Fenstergitter_v3 (Autodesk Fusion 360 design; units mm, degrees)
Autodesk Fusion 360 part; units mm, degrees
sketch "Skizze1" plane through (0, 0, 0) normal (0, 1, 0) x (1, 0, 0)
  line L0 (0, 0) -> (10, 0)
  line L1 (10, 0) -> (10, 28.5)
  line L2 (10, 28.5) -> (0, 28.5)
  line L3 (0, 28.5) -> (0, 0)
  line L4 (3.5, 9.5) -> (3.5, 3.5)
  arc A0 (3.5, 3.5) -> (6.5, 3.5) centre (5, 3.5) ccw
  line L5 (6.5, 3.5) -> (6.5, 9.5)
  arc A1 (6.5, 9.5) -> (3.5, 9.5) centre (5, 9.5) ccw
  line L6 (3.5, 21.5) -> (3.5, 15.5)
  line L7 (6.5, 15.5) -> (6.5, 21.5)
  arc A2 (6.5, 21.5) -> (3.5, 21.5) centre (5, 21.5) ccw
  arc A3 (3.5, 15.5) -> (6.5, 15.5) centre (5, 15.5) ccw
  dimension "d1" = 10
  dimension "d2" = 28.5
  dimension "d3" = 3
  dimension "d4" = 6
  dimension "d5" = 5
  dimension "d6" = 3.5
  dimension "d7" = 3
  dimension "d8" = 6
  dimension "d9" = 12
  constraint horizontal L0
  constraint vertical L1
  constraint horizontal L2
  constraint vertical L3
  constraint coincident L0.start L3.end
  constraint vertical L4
  constraint tangent L4 A0
  constraint tangent A0 L5
  constraint parallel L4 L5
  constraint tangent L5 A1
  constraint tangent L4 A1
  constraint vertical L6
  constraint tangent L6 A3
  constraint tangent L7 A3
  constraint parallel L6 L7
  constraint tangent L7 A2
  constraint tangent L6 A2
  measures "d1" distance of L0.start L0.end
  measures "d2" distance of L0.start L2.end
  measures "d3" distance of L4 L5
  measures "d4" distance of A0.centre A1.centre
  measures "d5" horizontal distance of L0.start A0.centre
  measures "d6" distance of L0 A0.centre
  measures "d7" distance of L6 L7
  measures "d8" distance of A3.centre A2.centre
  measures "d9" distance of A0.centre A3.centre
extrude "Extrusion1" add sketch "Skizze1" along normal blind 2
sketch "Skizze2" plane through (0, 2, 0) normal (0, 1, 0) x (-1, 0, 0)
  arc A0 (-6.5, -9.5) -> (-3.5, -9.5) centre (-5, -9.5) ccw
  line L0 (-6.5, -9.5) -> (-6.5, -3.5)
  arc A1 (-3.5, -3.5) -> (-6.5, -3.5) centre (-5, -3.5) ccw
  line L1 (-3.5, -3.5) -> (-3.5, -9.5)
  arc A2 (-3.5, -15.5) -> (-6.5, -15.5) centre (-5, -15.5) ccw
  line L2 (-3.5, -15.5) -> (-3.5, -21.5)
  arc A3 (-6.5, -21.5) -> (-3.5, -21.5) centre (-5, -21.5) ccw
  line L3 (-6.5, -21.5) -> (-6.5, -15.5)
  line L4 (0, -28.5) -> (0, 0)
  line L5 (0, 0) -> (-10, 0)
  line L6 (-10, 0) -> (-10, -28.5)
  line L7 (-10, -28.5) -> (0, -28.5)
  line L8 (-10, -28.5) -> (0, -28.5)
  line L9 (0, -28.5) -> (0, -25)
  line L10 (0, -25) -> (-10, -25)
  line L11 (-10, -25) -> (-10, -28.5)
  constraint horizontal L8
  constraint vertical L9
  constraint horizontal L10
  constraint vertical L11
  constraint coincident L4 L9.end
  constraint coincident L6.end L7.start
ref_plane "Arbeitsebene1" through (5, 18, -26.75) normal (0, 1, 0) x (-1, 0, 0)
sketch "Skizze3" plane through (5, 18, -26.75) normal (0, 1, 0) x (1, 0, 0)
ref_plane "Arbeitsebene2" through (5, 16, -6.5) normal (0, 1, 0) x (-1, 0, 0)
sketch "Skizze4" plane through (5, 16, -26.75) normal (0, 1, 0) x (1, 0, 0)
  arc A0 (1.5, -17.25) -> (-1.5, -17.25) centre (0, -17.25) ccw
  line L0 (1.5, -17.25) -> (1.5, -23.25)
  arc A1 (-1.5, -23.25) -> (1.5, -23.25) centre (0, -23.25) ccw
  line L1 (-1.5, -23.25) -> (-1.5, -17.25)
  arc A2 (-1.5, -11.25) -> (1.5, -11.25) centre (0, -11.25) ccw
  line L2 (-1.5, -11.25) -> (-1.5, -5.25)
  arc A3 (1.5, -5.25) -> (-1.5, -5.25) centre (0, -5.25) ccw
  line L3 (1.5, -5.25) -> (1.5, -11.25)
  line L4 (-5, 1.75) -> (-5, -26.75)
  line L5 (-5, -26.75) -> (5, -26.75)
  line L6 (5, -26.75) -> (5, 1.75)
  line L7 (5, 1.75) -> (-5, 1.75)
  line L8 (5, 1.75) -> (-5, 1.75)
  line L9 (-5, 1.75) -> (-5, -0.75)
  line L10 (-5, -0.75) -> (5, -0.75)
  line L11 (5, -0.75) -> (5, 1.75)
  dimension "d14" = 2.5
  constraint horizontal L8
  constraint vertical L9
  constraint horizontal L10
  constraint vertical L11
  constraint coincident L6.end L7.start
  measures "d14" distance of L6.end L10.end
loft "Erhebung1" add profiles "Skizze2", "Skizze4" section 1 contours L4 L6 L7 L8 L9 L10 L11 section 2 contours L4 L6 L7 L8 L9 L10 L11
sketch "Skizze5" plane through (0, 16, 0) normal (0, 1, 0) x (-1, 0, 0)
  line L0 (-10, -26) -> (-10, -28.5)
  line L1 (-10, -28.5) -> (0, -28.5)
  line L2 (0, -28.5) -> (0, -26)
  line L3 (0, -26) -> (-10, -26)
  line L4 (-10, -26) -> (0, -26)
  line L5 (0, -26) -> (0, -46)
  line L6 (0, -46) -> (-10, -46)
  line L7 (-10, -46) -> (-10, -26)
  dimension "d15" = 20
  constraint horizontal L4
  constraint vertical L5
  constraint horizontal L6
  constraint vertical L7
  constraint coincident L0.start L3.end
  measures "d15" distance of L0.start L6.end
extrude "Extrusion2" add sketch "Skizze5" along normal blind 1.2
fillet "Abrundung1" radius 0.3 19 faces at (4.9626, 0, -26.6653) (10, 6, -27.3333) (3.5, 0.6667, -19.5) (4.0075, 0.6667, -22.6247) (6.5, 0.6667, -17.5) (6.4095, 1.3333, -14.987) (4.3831, 1.3333, -2.1327) (3.5, 0.6667, -7.5) (3.5075, 1.3333, -9.6494) (6.5, 0.6667, -5.5) (6.6667, 6.6667, -25.3333) (1.1723, 2, -13.4255) (3.3333, 1.3333, 0) (3.3333, 16.4, -46) (0, 6, -27.3333) (3.3333, 16.4, -26) (6.6667, 16, -34.3333) (6.6667, 10.6667, -28.5) (6.6667, 17.2, -32.6667)
